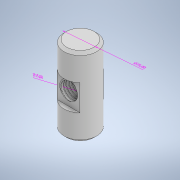
# Autodesk Inventor part: Pino Plataforma Deslizante
Saved by Autodesk Inventor 2021 (Build 250183000, 183)
## iProperties
Created: 2021-08-18
Part Number: Pino Plataforma Deslizante
Material: Generic
Document SubType Name: Modeling
Designer: guilh
Density: 1 g/cm^3
Appearance: Default
Author: guilh
Autodesk Inventor part; units mm, degrees
ref_plane "YZ Plane" through (0, 0, 0) normal (1, 0, 0) x (0, 1, 0)
ref_plane "XZ Plane" through (0, 0, 0) normal (0, 1, 0) x (-1, 0, 0)
ref_plane "XY Plane" through (0, 0, 0) normal (0, 0, 1) x (1, 0, 0)
sketch "Sketch1" plane through (0, 0, 0) normal (0, 1, 0) x (-1, 0, 0)
  circle A0 centre (0, 0) radius 12.5
  dimension "d0" = 25
  constraints: 1 centre point, 1 coincident
  measures "d0" diameter of A0
extrude "Extrusion1" add sketch "Sketch1" along normal blind 60
sketch "Sketch2" plane through (0, 0, 0) normal (0, 0, 1) x (1, 0, 0)
  line L0 (0, 0) -> (0, 30)
  circle A0 centre (0, 30) radius 7.5
  dimension "d3" = 30
  dimension "d4" = 15
  constraints: 2 end point, 1 centre point, 1 coincident, 1 vertical
  measures "d3" distance of L0.start L0.end
  measures "d4" diameter of A0
extrude "Extrusion2" cut sketch "Sketch2" along normal mid plane 60
chamfer "Chamfer1" distance 2 angle 45 2 edges at (12.5, 60, 0) (12.5, 0, 0)
sketch "Sketch3" plane through (0, 0, 0) normal (1, 0, 0) x (0, 1, 0)
  line L0 (0, 0) -> (20, 0)
  line L1 (20, 0) -> (20, -9)
  line L2 (2, -12.5) -> (58, -12.5) projected
  line L3 (20, -9) -> (40, -9)
  line L4 (40, -9) -> (40, 9)
  line L5 (40, 9) -> (20, 9)
  line L6 (20, 9) -> (20, 0)
  line L7 (40, -9) -> (40, -15.8527)
  line L8 (40, -15.8527) -> (20, -15.8527)
  line L9 (20, -15.8527) -> (20, -9)
  line L10 (20, 9) -> (20, 19.7516)
  line L11 (20, 19.7516) -> (40, 19.7516)
  line L12 (40, 19.7516) -> (40, 9)
  dimension "d20" = 20
  dimension "d21" = 9
  dimension "d22" = 20
  dimension "d23" = 18
  constraints: 24 end point, 7 perpendicular, 3 point on line, 2 collinear, 1 horizontal, 1 vertical
  measures "d20" distance of L0.start L0.end
  measures "d21" distance of L0.end L1.end
  measures "d22" distance of L1.end L3.end
  measures "d23" distance of L3.end L4.end
extrude "Extrusion3" cut sketch "Sketch3" along normal mid plane 25 contours L3 L7 L2 L9 | L10 L11 L12 L5 | L2 L7 L8 L9
sketch "Sketch5" plane through (-8.6747, 40, 9) normal (0, 0, 1) x (1, 0, 0)
  circle A0 centre (8.6747, -10) radius 7.5 projected
  circle A1 centre (8.6747, -10) radius 7.5
  circle A2 centre (8.6747, -10) radius 6.4175
  point P0 (8.6747, -40)
  dimension "d30" = 15
  dimension "d31" = 12.835
  constraints: 2 centre point, 2 coincident
  measures "d30" diameter of A1
  measures "d31" diameter of A2
extrude "Extrusion4" add sketch "Sketch5" against normal blind 18
sketch "Sketch6" plane through (0, 0, 0) normal (1, 0, 0) x (0, 1, 0)
  line L0 (0, 0) -> (0, -9)
  line L1 (0, -10.5) -> (0, 10.5) projected
  line L2 (40, -9) -> (20, -9) projected
  line L3 (36.4175, -9) -> (23.5825, -9) projected
  line L4 (0, -9) -> (23.5825, -9)
  line L5 (23.5825, -9) -> (23.5825, -11)
  line L6 (23.5825, -11) -> (23.5825, -10)
  line L7 (30, -9) -> (22.41, -9)
  line L8 (22.41, -9) -> (22.41, -10)
  line L9 (22.41, -10) -> (22.536, -10)
  arc A0 (22.41, -10) -> (22.473, -10.1091) centre (22.536, -10) ccw
  line L10 (22.536, -10) -> (22.473, -10.1091) construction
  line L11 (22.536, -10) -> (22.41, -10) construction
  arc A1 (22.473, -9.8909) -> (22.41, -10) centre (22.536, -10) ccw
  line L12 (22.536, -10) -> (22.473, -9.8909) construction
  line L13 (22.536, -10) -> (22.41, -10) construction
  line L14 (22.473, -9.8909) -> (23.5825, -9.2503)
  line L15 (22.473, -10.1091) -> (23.5825, -10.7497)
  dimension "d34" = 9
  dimension "d37" = 1
  dimension "d40" = 1
  dimension "d41" = 0.126
  dimension "d42" = 60
  dimension "d43" = 60
  constraints: 26 end point, 4 point on circle, 4 point on line, 2 centre point, 2 coincident, 2 midpoint, 1 horizontal, 1 perpendicular, 1 vertical
  measures "d34" distance of L0.start L0.end
  measures "d37" distance of L5.end L6.end
  measures "d40" distance of L7.end L8.end
  measures "d41" distance of L8.end L9.end
  measures "d42" angle of L11 L10
  measures "d43" angle of L12 L13
sketch "Sketch7" plane through (0, 0, 0) normal (1, 0, 0) x (0, 1, 0)
  line L0 (40, -9) -> (20, -9) projected
  line L1 (30, -9) -> (30, 9)
  point P0 (0, 0)
  dimension "d44" = 18
  constraints: 2 end point, 1 midpoint, 1 vertical
  measures "d44" distance of L1.start L1.end
coil "Coil1" sketch "Sketch6" operation cut axis through (0, 30, -9) along (0, 0, 1) pitch 2 turns 10 hand right contours L5 L15 A0 A1 L14
body "Solid1"
